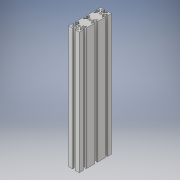
# Autodesk Inventor part: 1545rail_17inch
Saved by Autodesk Inventor 2018 (Build 220112000, 112)
## iProperties
Created: 2020-03-10
Part Number: 1545rail_17inch
Material: Generic
Document SubType Name: Modeling
Designer: natha
Density: 1 g/cm^3
Appearance: Default
Author: natha
Autodesk Inventor part; units mm, degrees
ref_plane "YZ Plane" through (0, 0, 0) normal (1, 0, 0) x (0, 1, 0)
ref_plane "XZ Plane" through (0, 0, 0) normal (0, 1, 0) x (-1, 0, 0)
ref_plane "XY Plane" through (0, 0, 0) normal (0, 0, 1) x (1, 0, 0)
sketch "Sketch1" plane through (0, 0, 0) normal (0, 1, 0) x (-1, 0, 0)
  circle A0 centre (19.05, -19.05) radius 3.3274
  circle A1 centre (19.05, -57.15) radius 3.3274
  circle A2 centre (19.05, -95.25) radius 3.3274
  line L0 (0, 0) -> (15.0114, 0)
  line L1 (15.0114, 0) -> (15.0114, -4.2672)
  line L2 (15.0114, -4.2672) -> (8.001, -4.2672)
  line L3 (38.1, 0) -> (23.0886, 0)
  line L4 (23.0886, 0) -> (23.0886, -4.2672)
  line L5 (23.0886, -4.2672) -> (30.099, -4.2672)
  line L6 (8.001, -4.2672) -> (15.0114, -11.9888)
  line L7 (30.099, -4.2672) -> (23.0886, -11.9888)
  line L8 (23.0886, -11.9888) -> (15.0114, -11.9888)
  line L9 (38.1, 0) -> (38.1, -15.0114)
  line L10 (38.1, -15.0114) -> (33.8328, -15.0114)
  line L11 (33.8328, -15.0114) -> (33.8328, -8.001)
  line L12 (26.1112, -15.0114) -> (26.1112, -25.8654)
  line L13 (33.8328, -8.001) -> (26.1112, -15.0114)
  line L14 (38.1, -24.6888) -> (33.8328, -24.6888)
  line L15 (33.8328, -24.6888) -> (33.8328, -31.6992)
  line L16 (33.8328, -31.6992) -> (26.1112, -25.8654)
  line L17 (38.1, -114.3) -> (38.1, -99.2886)
  line L18 (38.1, -99.2886) -> (33.8328, -99.2886)
  line L19 (33.8328, -99.2886) -> (33.8328, -106.299)
  line L20 (38.1, -114.3) -> (23.0886, -114.3)
  line L21 (23.0886, -114.3) -> (23.0886, -110.0328)
  line L22 (23.0886, -110.0328) -> (30.099, -110.0328)
  line L23 (0, -114.3) -> (15.0114, -114.3)
  line L24 (15.0114, -114.3) -> (15.0114, -110.0328)
  line L25 (15.0114, -110.0328) -> (8.001, -110.0328)
  line L26 (23.0886, -102.3112) -> (15.0114, -102.3112)
  line L27 (23.0886, -102.3112) -> (30.099, -110.0328)
  line L28 (15.0114, -102.3112) -> (8.001, -110.0328)
  line L29 (38.1, -24.6888) -> (38.1, -54.1528)
  line L30 (38.1, -54.1528) -> (33.8328, -54.1528)
  line L31 (33.8328, -54.1528) -> (33.8328, -47.1424)
  line L32 (26.1112, -54.6354) -> (26.1112, -62.7126)
  line L33 (33.8328, -47.1424) -> (26.1112, -54.6354)
  line L34 (38.1, -62.7126) -> (33.8328, -62.7126)
  line L35 (33.8328, -62.7126) -> (33.8328, -69.723)
  line L36 (33.8328, -69.723) -> (26.1112, -62.7126)
  line L37 (38.1, -91.9226) -> (33.8328, -91.9226)
  line L38 (33.8328, -91.9226) -> (33.8328, -84.9122)
  line L39 (38.1, -62.7126) -> (38.1, -91.9226)
  line L40 (28.0178, -91.9226) -> (28.0178, -99.2886)
  line L41 (28.0178, -99.2886) -> (33.8328, -106.299)
  line L42 (33.8328, -84.9122) -> (28.0178, -91.9226)
  line L43 (11.9888, -54.6354) -> (11.9888, -62.7126)
  line L44 (11.9888, -93.3774) -> (11.9888, -99.2886)
  line L45 (0, 0) -> (0, -15.0114)
  line L46 (0, -15.0114) -> (4.2672, -15.0114)
  line L47 (4.2672, -15.0114) -> (4.2672, -8.001)
  line L48 (11.9888, -15.7226) -> (11.9888, -25.8654)
  line L49 (4.2672, -8.001) -> (11.9888, -15.7226)
  line L50 (0, -114.3) -> (0, -99.2886)
  line L51 (0, -99.2886) -> (4.2672, -99.2886)
  line L52 (4.2672, -99.2886) -> (4.2672, -106.299)
  line L53 (4.2672, -106.299) -> (11.9888, -99.2886)
  line L54 (0, -63.9406) -> (0, -93.1506)
  line L55 (0, -93.1506) -> (4.2672, -93.1506)
  line L56 (4.2672, -93.1506) -> (4.2672, -86.1402)
  line L57 (4.2672, -86.1402) -> (11.9888, -93.3774)
  line L58 (0, -63.9406) -> (4.2672, -63.9406)
  line L59 (4.2672, -63.9406) -> (4.2672, -70.951)
  line L60 (4.2672, -70.951) -> (11.9888, -62.7126)
  line L61 (0, -55.2632) -> (0, -24.6888)
  line L62 (0, -24.6888) -> (4.5476, -24.6888)
  line L63 (4.5476, -24.6888) -> (4.5476, -31.6992)
  line L64 (4.5476, -31.6992) -> (11.9888, -25.8654)
  line L65 (0, -55.2632) -> (4.2672, -55.2632)
  line L66 (4.2672, -55.2632) -> (4.2672, -48.2528)
  line L67 (4.2672, -48.2528) -> (11.9888, -54.6354)
  dimension "d0" = 38.1
  dimension "d1" = 114.3
  dimension "d2" = 6.6548
  dimension "d3" = 6.6548
  dimension "d4" = 6.6548
  dimension "d11" = 15.0114
  dimension "d12" = 4.2672
  dimension "d14" = 15.0114
  dimension "d15" = 7.0104
  dimension "d19" = 15.0114
  dimension "d20" = 4.2672
  dimension "d21" = 7.0104
  dimension "d22" = 11.9888
  dimension "d23" = 4.2672
  dimension "d24" = 7.0104
  dimension "d25" = 9.6774
  dimension "d26" = 15.0114
  dimension "d27" = 7.0104
  dimension "d28" = 15.0114
  dimension "d29" = 4.2672
  dimension "d30" = 7.0104
  dimension "d31" = 15.0114
  dimension "d32" = 7.0104
  dimension "d33" = 11.9888
  dimension "d34" = 29.464
  dimension "d35" = 7.0104
  dimension "d36" = 8.0772
  dimension "d37" = 11.9888
  dimension "d38" = 7.0104
  dimension "d39" = 7.0104
  dimension "d40" = 15.0114
  dimension "d41" = 4.2672
  dimension "d42" = 7.0104
  dimension "d43" = 11.9888
  dimension "d44" = 11.9888
  dimension "d45" = 11.9888
  dimension "d46" = 15.0114
  dimension "d47" = 4.2672
  dimension "d48" = 7.0104
  dimension "d49" = 7.0104
  dimension "d50" = 4.2672
  dimension "d51" = 7.0104
  dimension "d52" = 29.21
  dimension "d53" = 29.21
  dimension "d54" = 7.0104
  dimension "d55" = 4.2672
  dimension "d56" = 7.0104
  constraints: 136 end point, 26 perpendicular, 13 vertical, 9 horizontal, 8 point on line, 3 centre point
  measures "d0" distance of L17.start L23.start
  measures "d1" distance of L3.start L17.start
  measures "d2" diameter of A0
  measures "d3" diameter of A1
  measures "d4" diameter of A2
  measures "d11" distance of L0.start L0.end
  measures "d12" distance of L0.end L1.end
  measures "d14" distance of L3.start L3.end
  measures "d15" distance of L4.end L5.end
  measures "d19" distance of L3.start L9.end
  measures "d20" distance of L9.end L10.end
  measures "d21" distance of L10.end L11.end
  measures "d22" distance between parallel lines of L12 L9
  measures "d23" distance of L14.start L14.end
  measures "d24" distance of L14.end L15.end
  measures "d25" distance between parallel lines of L14 L10
  measures "d26" distance of L17.start L17.end
  measures "d27" distance of L18.end L19.end
  measures "d28" distance of L17.start L20.end
  measures "d29" distance of L20.end L21.end
  measures "d30" distance of L21.end L22.end
  measures "d31" distance of L23.start L23.end
  measures "d32" distance of L24.end L25.end
  measures "d33" distance between parallel lines of L20 L26
  measures "d34" distance of L14.start L29.end
  measures "d35" distance of L30.end L31.end
  measures "d36" distance of L32.start L32.end
  measures "d37" distance between parallel lines of L32 L29
  measures "d38" distance of L34.end L35.end
  measures "d39" distance of L37.end L38.end
  measures "d40" distance of L0.start L45.end
  measures "d41" distance of L45.end L46.end
  measures "d42" distance of L46.end L47.end
  measures "d43" distance between parallel lines of L45 L48
  measures "d44" distance between parallel lines of L45 L43
  measures "d45" distance between parallel lines of L45 L44
  measures "d46" distance of L23.start L50.end
  measures "d47" distance of L50.end L51.end
  measures "d48" distance of L51.end L52.end
  measures "d49" distance of L55.end L56.end
  measures "d50" distance of L54.start L58.end
  measures "d51" distance of L58.end L59.end
  measures "d52" distance of L34.start L37.start
  measures "d53" distance of L54.start L54.end
  measures "d54" distance of L62.end L63.end
  measures "d55" distance of L61.start L65.end
  measures "d56" distance of L65.end L66.end
extrude "Extrusion1" add sketch "Sketch1" along normal blind 431.8
body "Solid1"
